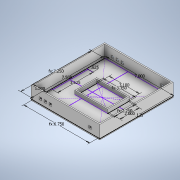
# Autodesk Inventor part: RCcar_full build
Saved by Autodesk Inventor 2022 (Build 260153000, 153)
## iProperties
Created: 2022-03-25
Part Number: RCcar_full build
Material: Generic
Document SubType Name: Modeling
Designer: saipr
Density: 1 g/cm^3
Appearance: Default
Author: saipr
Autodesk Inventor part; units mm, degrees
ref_plane "YZ Plane" through (0, 0, 0) normal (1, 0, 0) x (0, 1, 0)
ref_plane "XZ Plane" through (0, 0, 0) normal (0, 1, 0) x (-1, 0, 0)
ref_plane "XY Plane" through (0, 0, 0) normal (0, 0, 1) x (1, 0, 0)
sketch "Sketch1" plane through (0, 0, 0) normal (0, 1, 0) x (-1, 0, 0)
  line L0 (0, 0) -> (177.8, 0)
  line L1 (177.8, 0) -> (177.8, -190.5)
  line L2 (177.8, -190.5) -> (0, -190.5)
  line L3 (0, -190.5) -> (0, 0)
  line L4 (114.3, -3.175) -> (114.3, -187.325)
  line L5 (174.625, -93.6625) -> (3.175, -96.8375)
  line L6 (128.27, -69.85) -> (49.53, -69.85)
  line L7 (49.53, -69.85) -> (49.53, -120.65)
  line L8 (49.53, -120.65) -> (128.27, -120.65)
  line L9 (128.27, -120.65) -> (128.27, -69.85)
  line L10 (128.27, -69.85) -> (49.53, -120.65) construction
  line L11 (49.53, -69.85) -> (128.27, -120.65) construction
  line L12 (131.445, -66.675) -> (46.355, -66.675)
  line L13 (46.355, -66.675) -> (46.355, -123.825)
  line L14 (46.355, -123.825) -> (131.445, -123.825)
  line L15 (131.445, -123.825) -> (131.445, -66.675)
  line L16 (131.445, -66.675) -> (46.355, -123.825) construction
  line L17 (46.355, -66.675) -> (131.445, -123.825) construction
  line L18 (3.175, -187.325) -> (174.625, -187.325)
  line L19 (174.625, -187.325) -> (174.625, -3.175)
  line L20 (174.625, -3.175) -> (3.175, -3.175)
  line L21 (3.175, -3.175) -> (3.175, -187.325)
  line L22 (3.175, -187.325) -> (174.625, -3.175) construction
  line L23 (174.625, -187.325) -> (3.175, -3.175) construction
  line L24 (174.625, -93.6625) -> (174.625, -187.325)
  line L25 (174.625, -140.4938) -> (158.75, -140.4938)
  line L26 (174.625, -93.6625) -> (174.625, -3.175)
  line L27 (174.625, -48.4188) -> (209.55, -48.4188)
  line L28 (209.55, -48.4188) -> (171.45, -48.4188)
  line L29 (171.45, -48.4188) -> (171.45, -140.4938)
  line L30 (171.45, -140.4938) -> (158.75, -140.4938)
  point P0 (88.9, -95.25)
  point P1 (88.9, -95.25)
  dimension "d0" = 177.8
  dimension "d1" = 190.5
  dimension "d2" = 78.74
  dimension "d3" = 50.8
  dimension "d4" = 85.09
  dimension "d5" = 57.15
  dimension "d6" = 171.45
  dimension "d7" = 184.15
  dimension "d18" = 15.875
  dimension "d22" = 38.1
  dimension "d23" = 92.075
  dimension "d48" = 3.175
  constraints: 62 end point, 10 midpoint, 8 parallel, 6 horizontal, 5 perpendicular, 5 point on line, 2 collinear
  measures "d0" distance of L1.end L2.end
  measures "d1" distance of L0.end L1.end
  measures "d2" distance of L8.end L7.end
  measures "d3" distance of L7.end L6.end
  measures "d4" distance of L14.end L13.end
  measures "d5" distance of L13.end L12.end
  measures "d6" distance of L20.end L19.end
  measures "d7" distance of L19.end L18.end
  measures "d18" distance of L25.start L25.end
  measures "d22" distance of L27.end L28.end
  measures "d23" distance of L28.end L29.end
  measures "d48" distance between parallel lines of L3 L21
extrude "Extrusion1" add sketch "Sketch1" against normal blind 3.175 contours L0 L1 L2 L3 | L20 L19 L28 L29 L5 L15 L12 L4 | L4 L12 L13 L5 L21 L20 | L12 L15 L5 L9 L6 L4 | L4 L6 L7 L5 L13 L12 | L6 L9 L5 L4 | L4 L5 L7 L6 | L19 L5 L29 L28 | L5 L13 L14 L4 L18 L21 | L5 L9 L8 L4 | L4 L8 L7 L5 | L15 L14 L4 L8 L9 L5 | L5 L29 L25 L19 L18 L4 L14 L15 | L5 L7 L8 L4 L14 L13 | L19 L25 L29 L5
extrude "Extrusion2" add sketch "Sketch1" along normal blind 9.525 contours L12 L15 L5 L9 L6 L4 | L4 L6 L7 L5 L13 L12 | L6 L9 L5 L4 | L4 L5 L7 L6 | L5 L9 L8 L4 | L4 L8 L7 L5 | L15 L14 L4 L8 L9 L5 | L5 L7 L8 L4 L14 L13
extrude "Extrusion3" cut sketch "Sketch1" along normal blind 9.525 contours L6 L9 L5 L4 | L4 L5 L7 L6 | L5 L9 L8 L4 | L4 L8 L7 L5
extrude "Extrusion4" cut sketch "Sketch1" along normal blind 9.525 contours L6 L9 L5 L4 | L4 L5 L7 L6 | L5 L9 L8 L4 | L4 L8 L7 L5
extrude "Extrusion5" add sketch "Sketch1" along normal blind 31.75
sketch "Sketch2" plane through (0, -3.175, -190.5) normal (0, 0, -1) x (-1, 0, 0)
  line L0 (177.8, 34.925) -> (177.8, 0) projected
  line L1 (177.8, 34.925) -> (123.825, 34.925)
  line L2 (123.825, 34.925) -> (123.825, 0)
  line L3 (0, 0) -> (177.8, 0) projected
  line L4 (177.8, 0) -> (177.8, 15.875)
  line L5 (177.8, 15.875) -> (123.825, 15.875)
  line L6 (177.8, 15.875) -> (153.9875, 15.875)
  line L7 (153.9875, 15.875) -> (141.2875, 15.875)
  line L8 (150.8125, 12.7) -> (157.1625, 12.7)
  line L9 (157.1625, 12.7) -> (157.1625, 19.05)
  line L10 (157.1625, 19.05) -> (150.8125, 19.05)
  line L11 (150.8125, 19.05) -> (150.8125, 12.7)
  line L12 (150.8125, 12.7) -> (157.1625, 19.05) construction
  line L13 (157.1625, 12.7) -> (150.8125, 19.05) construction
  line L14 (144.4625, 12.7) -> (138.1125, 12.7)
  line L15 (138.1125, 12.7) -> (138.1125, 19.05)
  line L16 (138.1125, 19.05) -> (144.4625, 19.05)
  line L17 (144.4625, 19.05) -> (144.4625, 12.7)
  line L18 (144.4625, 12.7) -> (138.1125, 19.05) construction
  line L19 (138.1125, 12.7) -> (144.4625, 19.05) construction
  line L20 (141.2875, 15.875) -> (127, 15.875)
  line L21 (127, 15.875) -> (25.4, 15.875)
  line L22 (141.2875, 15.875) -> (128.5875, 15.875)
  line L23 (125.4125, 12.7) -> (131.7625, 12.7)
  line L24 (131.7625, 12.7) -> (131.7625, 19.05)
  line L25 (131.7625, 19.05) -> (125.4125, 19.05)
  line L26 (125.4125, 19.05) -> (125.4125, 12.7)
  line L27 (125.4125, 12.7) -> (131.7625, 19.05) construction
  line L28 (131.7625, 12.7) -> (125.4125, 19.05) construction
  line L29 (22.225, 19.05) -> (28.575, 19.05)
  line L30 (28.575, 19.05) -> (28.575, 12.7)
  line L31 (28.575, 12.7) -> (22.225, 12.7)
  line L32 (22.225, 12.7) -> (22.225, 19.05)
  line L33 (22.225, 19.05) -> (28.575, 12.7) construction
  line L34 (28.575, 19.05) -> (22.225, 12.7) construction
  line L35 (0, 0) -> (0, 34.925) projected
  point P0 (0, 3.175)
  dimension "d25" = 15.875
  dimension "d27" = 12.7
  dimension "d28" = 6.35
  dimension "d29" = 6.35
  dimension "d30" = 6.35
  dimension "d31" = 6.35
  dimension "d32" = 14.2875
  dimension "d36" = 101.6
  dimension "d38" = 12.7
  dimension "d39" = 6.35
  dimension "d40" = 6.35
  dimension "d41" = 6.35
  dimension "d42" = 6.35
  dimension "d44" = 25.4
  dimension "d45" = 53.975
  constraints: 66 end point, 8 midpoint, 8 parallel, 7 point on line, 6 horizontal, 5 perpendicular, 1 coincident, 1 vertical
  measures "d25" distance of L0.end L4.end
  measures "d27" distance of L6.end L7.end
  measures "d28" distance of L10.end L9.end
  measures "d29" distance of L9.end L8.end
  measures "d30" distance of L15.end L16.end
  measures "d31" distance of L14.end L15.end
  measures "d32" distance of L7.end L20.end
  measures "d36" distance of L21.start L21.end
  measures "d38" distance of L7.end L22.end
  measures "d39" distance of L25.end L24.end
  measures "d40" distance of L24.end L23.end
  measures "d41" distance of L30.end L31.end
  measures "d42" distance of L29.end L30.end
  measures "d44" distance from line of L35 L21.end
  measures "d45" distance between parallel lines of L2 L0
extrude "Extrusion6" cut sketch "Sketch2" against normal blind 190.5 contours L9 L8 L11 L5 | L5 L11 L10 L9 | L26 L25 L24 L5 | L5 L24 L23 L26 | L17 L14 L15 L5 | L5 L15 L16 L17 | L29 L30 L31 L32
body "Solid1"
